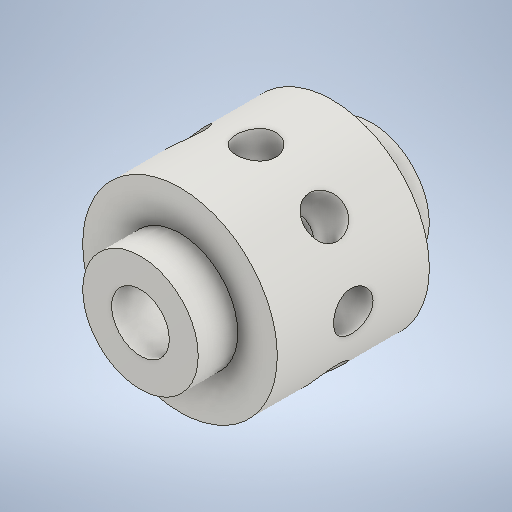
# Autodesk Inventor part: 13A FLYWHEEL HUB
Saved by Autodesk Inventor 2025.2 (Build 292293000, 293)
## iProperties
Created: 2025-05-29
Part Number: 13A FLYWHEEL HUB
Material: Steel AISI 1020 107 HR
Document SubType Name: Modeling
Designer: bless
Density: 7.87 g/cm^3
Appearance: Steel
Author: bless
Autodesk Inventor part; units mm, degrees
ref_plane "XZ Plane" through (0, 0, 0) normal (0, 1, 0) x (-1, 0, 0)
ref_plane "XY Plane" through (0, 0, 0) normal (0, 0, 1) x (1, 0, 0)
sketch "Sketch1" plane through (0, 0, 0) normal (0, 0, 1) x (1, 0, 0)
  circle A0 centre (0, 0) radius 9.5
  dimension "d0" = 19
  constraints: 1 centre point, 1 coincident
  measures "d0" diameter of A0
extrude "Extrusion1" add sketch "Sketch1" along normal blind 6.5
sketch "Sketch2" plane through (0, 0, 0) normal (0, 0, -1) x (-1, 0, 0)
  circle A0 centre (0, 0) radius 9.5 projected
  circle A1 centre (0, 0) radius 16
  dimension "d3" = 32
  constraints: 1 centre point, 1 coincident
  measures "d3" diameter of A1
extrude "Extrusion2" add sketch "Sketch2" along normal blind 25 contours A0 | A1
sketch "Sketch3" plane through (0, 0, -25) normal (0, 0, -1) x (-1, 0, 0)
  circle A0 centre (0, 0) radius 16 projected
  circle A1 centre (0, 0) radius 9.5
  dimension "d6" = 19
  constraints: 1 centre point, 1 coincident
  measures "d6" diameter of A1
extrude "Extrusion3" add sketch "Sketch3" along normal blind 6.5 contours A1
sketch "Sketch4" plane through (0, 0, 0) normal (1, 0, 0) x (0, 1, 0)
  circle A0 centre (0, -28.4674) radius 1.5
  line L0 (9.5, 6.5) -> (-9.5, 6.5) projected
  point P0 (0, 0)
  dimension "d9" = 3
  dimension "d10" = 28.4674
  dimension "d11" = 34.9674
  constraints: 1 centre point
  measures "d9" diameter of A0
  measures "d10" distance of point (0, 0) A0.centre
  measures "d11" distance from line of L0 A0.centre
extrude "Extrusion4" cut sketch "Sketch4" along normal through all both and the other way through all
ref_plane "Work Plane1" through (16, 0, 0) normal (1, 0, 0) x (0, 1, 0)
sketch "Sketch5" plane through (16, 0, 0) normal (1, 0, 0) x (0, 1, 0)
  circle A0 centre (0, -12.5) radius 3.25
  line L0 (-9.5, -31.5) -> (9.5, -31.5) projected
  point P0 (0, 0)
  dimension "d15" = 6.5
  dimension "d16" = 19
  constraints: 1 centre point, 1 vertical alignment
  measures "d15" diameter of A0
  measures "d16" distance from line of L0 A0.centre
extrude "Extrusion5" cut sketch "Sketch5" against normal blind 8.17
pattern_circular "Circular Pattern1" count 8 over 360 about axis through (0, 0, -10) along (0, 0, 1) of "Extrusion5"
sketch "Sketch6" plane through (0, 0, 6.5) normal (0, 0, 1) x (1, 0, 0)
  circle A0 centre (0, 0) radius 9.5 projected
  circle A1 centre (0, 0) radius 4.75
  dimension "d22" = 9.5
  constraints: 1 centre point, 1 coincident
  measures "d22" diameter of A1
extrude "Extrusion6" cut sketch "Sketch6" against normal through all contours A1
body "Solid1"
